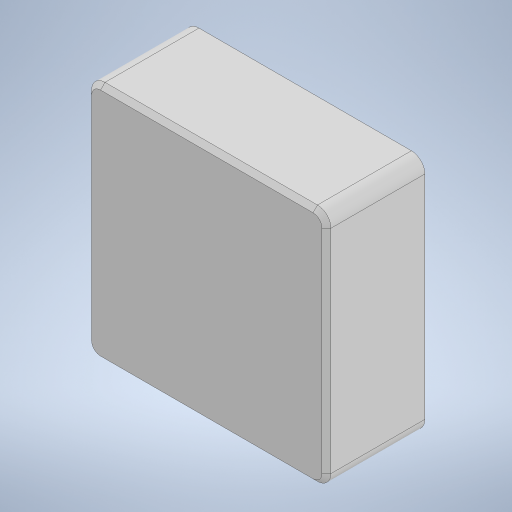
# Autodesk Inventor part: spodni_vlozka
Saved by Autodesk Inventor 2024 (Build 280153000, 153)
## iProperties
Created: 2024-03-13
Part Number: spodni_vlozka
Material: Všeobecné
Document SubType Name: Modeling
Designer: 42060
Density: 1 g/cm^3
Appearance: Výchozí
Author: 42060
Autodesk Inventor part; units mm, degrees
ref_plane "YZ Plane" through (0, 0, 0) normal (1, 0, 0) x (0, 1, 0)
ref_plane "XZ Plane" through (0, 0, 0) normal (0, 1, 0) x (-1, 0, 0)
ref_plane "XY Plane" through (0, 0, 0) normal (0, 0, 1) x (1, 0, 0)
sketch "Náčrt1" plane through (0, 0, 0) normal (0, 1, 0) x (-1, 0, 0)
  line L0 (49.5, 49.5) -> (-49.5, 49.5)
  line L1 (-49.5, 49.5) -> (-49.5, -49.5)
  line L2 (-49.5, -49.5) -> (49.5, -49.5)
  line L3 (49.5, -49.5) -> (49.5, 49.5)
  line L4 (49.5, 49.5) -> (-49.5, -49.5) construction
  line L5 (-49.5, 49.5) -> (49.5, -49.5) construction
  line L6 (53.5, 53.5) -> (-53.5, 53.5)
  line L7 (-53.5, 53.5) -> (-53.5, -53.5)
  line L8 (-53.5, -53.5) -> (53.5, -53.5)
  line L9 (53.5, -53.5) -> (53.5, 53.5)
  line L10 (53.5, 53.5) -> (-53.5, -53.5) construction
  line L11 (-53.5, 53.5) -> (53.5, -53.5) construction
  point P0 (0, 0)
  dimension "d1" = 99
  dimension "d4" = 4
  constraints: 24 end point, 4 midpoint, 4 parallel, 4 perpendicular, 2 horizontal
  measures "d1" distance of L0.end L1.end
  measures "d4" distance between parallel lines of L1 L7
extrude "Vysunutí1" add sketch "Náčrt1" along normal blind 44
extrude "Vysunutí2" add sketch "Náčrt1" along normal blind 5 contours L3 L2 L1 L0
fillet "Zaoblení1" radius 6 4 edges at (53.5, 22, 53.5) (53.5, 22, -53.5) (-53.5, 22, -53.5) (-53.5, 22, 53.5)
sketch "Náčrt2" plane through (-49.5, 44, 49.5) normal (1, 0, 0) x (0, 0, -1)
  circle A0 centre (82.5, -25) radius 16.5
  circle A1 centre (82.5, -25) radius 17.5
  line L0 (0, -39) -> (99, -39) projected
  line L1 (99, -39) -> (99, 0) projected
  point P0 (49.5, -44)
  point P1 (99, -44)
  point P2 (99, -44)
  point P3 (99, -44)
  dimension "d12" = 33
  dimension "d14" = 1
  dimension "d17" = 14
  constraints: 2 centre point, 1 tangent
  measures "d12" diameter of A0
  measures "d14" radial gap between concentric circles of A0 A1
  measures "d17" distance from line of L0 A0.centre
extrude "Vysunutí3" cut sketch "Náčrt2" along normal blind 26 contours A0 L0 | L1 A1 L0 A0 | L1 A1 | A0 L0 A1 L1 | L0 A0 | A0 L0 A1
fillet "Zaoblení3" radius 2.5 1 edges at (0, 5, -49.5)
fillet "Zaoblení4" radius 4 4 edges at (-36.5, 5, -22.5) (-36.5, 5, -43.5) (-36.5, 13.169, -49.5) (-36.5, 24.831, -49.5)
chamfer "Zkosení1" distance 0.5 angle 45 6 edges at (-23.5, 5, -44.129) (-23.5, 5, -33) (-23.5, 5, -21.871) (-23.5, 12.8442, -49.5) (-23.5, 19, -49.5) (-23.5, 25.1558, -49.5)
sketch "Náčrt3" plane through (-49.5, 44, 49.5) normal (1, 0, 0) x (0, 0, -1)
  line L0 (0, -39) -> (70.742, -39) projected
  line L1 (0, -39) -> (0, 0) projected
  line L2 (0, -39) -> (-0.75, -39)
  line L3 (-0.75, -39) -> (0.5897, -34)
  line L4 (0.5897, -34) -> (0, -33.4103)
  point P0 (49.5, -44)
  point P1 (0, -36.201)
  dimension "d23" = 75
  dimension "d24" = 0.75
  dimension "d25" = 5
  dimension "d26" = 120
  constraints: 6 end point, 1 horizontal, 1 point on line
  measures "d23" angle of L0 L3
  measures "d24" distance of L0.start L2.end
  measures "d25" distance from line of L0 L3.end
  measures "d26" angle of L3 L4
extrude "Vysunutí4" cut sketch "Náčrt3" along normal up to surface (99 mm away) contours L2 L3 L1
extrude "Vysunutí5" add sketch "Náčrt3" along normal up to surface (99 mm away) contours L1 L4 L3
chamfer "Zkosení2" distance 1 angle 45 4 edges at (0, 44, 49.5) (-49.5, 44, 0) (0, 44, -49.5) (49.5, 44, 0)
chamfer "Zkosení3" distance 2 angle 45 8 edges at (-53.5, 0, 0) (-51.7426, 0, 51.7426) (0, 0, 53.5) (51.7426, 0, 51.7426) (53.5, 0, 0) (51.7426, 0, -51.7426) (0, 0, -53.5) (-51.7426, 0, -51.7426)
mirror "Zrcadlit1" about plane through (0, 0, 0) normal (1, 0, 0) of "Vysunutí3", "Zaoblení4", "Zkosení1"
